# Autodesk Inventor part: ANSI L 3 x 2 x 3_16 00000012
Saved by Autodesk Inventor 2021 (Build 250183000, 183)
## iProperties
Created: 2008-01-07
Part Number: ANSI L 3 x 2 x 3_16 00000012
Material: Generic
Document SubType Name: Modeling
Standard: ANSI
Designer: nino.caldarola
Size Designation: L 3 x 2 x 3/16
Stock Number: L 3 x 2 x 3/16
Density: 1 g/cm^3
Appearance: Default
_FrameMemberDoc: Frame Member File
_Version: 12.0.0
_CCFamilyMember: 5
_CCFamilyDisplayName: ANSI L (Unequal angles) - Angle Steel
G_L: 14.738 in
G_W: 2.000 in
G_H: 3.000 in
+E866665F-DFCD-4B43-A752-D40B89ECAD35+CUTDETAIL1: Miter 67.50 deg
+05D53CF9-7399-4BD2-B0F9-E004F241F57C+CUTDETAIL2: Miter 67.50 deg
Author: nino.caldarola
Autodesk Inventor part; units mm, degrees
ref_plane "Start plane" through (0, 0, -21.042) normal (0, 0, 1) x (1, 0, 0)
ref_plane "End plane" through (0, 0, 353.3115) normal (0, 0, 1) x (1, 0, 0)
sketch "Sketch" plane through (0, 0, 0) normal (0, 0, 1) x (1, 0, 0)
  line L0 (0, 76.2) -> (0, 0)
  line L1 (0, 0) -> (50.8, 0)
  line L2 (50.8, 0) -> (50.8, 2.7625)
  line L3 (48.8, 4.7625) -> (12.6365, 4.7625)
  line L4 (4.7625, 12.6365) -> (4.7625, 74.2)
  line L5 (2.7625, 76.2) -> (0, 76.2)
  line L6 (-7.0414, 0) -> (21.5385, 0) construction
  line L7 (0, -8.0414) -> (0, 34.5385) construction
  arc A0 (4.7625, 12.6365) -> (12.6365, 4.7625) centre (12.6365, 12.6365) ccw
  arc A1 (50.8, 2.7625) -> (48.8, 4.7625) centre (48.8, 2.7625) ccw
  arc A2 (4.7625, 74.2) -> (2.7625, 76.2) centre (2.7625, 74.2) ccw
  line L8 (0, 93.5453) -> (0, -24.9725) construction
  line L9 (-18.6925, 0) -> (62.8653, 0) construction
  point P0 (50.8, 4.7625)
  point P1 (4.7625, 4.7625)
  point P2 (4.7625, 76.2)
  dimension "d12" = 4.7625
  dimension "d13" = 76.2
  dimension "d14" = 50.8
  dimension "d15" = 0
  dimension "d16" = 4.7625
  dimension "d17" = 0
  dimension "d18" = 7.874
  dimension "d19" = 2
  constraints: 16 end point, 6 point on circle, 6 point on line, 6 tangent, 3 centre point, 2 collinear, 2 parallel, 1 equal radius
  measures "d12" distance between parallel lines of L4 L0
  measures "d13" distance of L0.start L1.start
  measures "d14" distance of L1.start L1.end
  measures "d15" distance between parallel lines of L6 L1
  measures "d16" distance between parallel lines of L1 L3
  measures "d17" distance between parallel lines of L7 L0
  measures "d18" radius of A0
  measures "d19" radius of A1
extrude "Body" add sketch "Sketch" along normal up to surface (374.3536 mm away) from surface at -21.042
ref_plane "Work Plane3" through (50.8, 38.1, -21.042) normal (-0.3827, 0, -0.9239) x (-0.9239, 0, 0.3827)
split "Split1" plane through (50.8, 38.1, -21.042) removes the side toward (-0.3827, 0, -0.9239)
ref_plane "Work Plane4" through (50.8, 38.1, 353.3115) normal (-0.3827, 0, 0.9239) x (0.9239, 0, 0.3827)
split "Split2" plane through (50.8, 38.1, 353.3115) removes the side toward (-0.3827, 0, 0.9239)
equation "\"d12\" = G_T"
equation "\"d13\" = G_H"
equation "\"d14\" = G_W"
equation "\"d16\" = G_T"
equation "\"d18\" = G_IR"
equation "\"d4\" = G_L"
equation "\"G_W\" = 50.8"
equation "\"G_H\" = 76.2"
equation "\"G_T\" = 4.7625"
equation "\"G_ER\" = 4.064"
equation "\"G_IR\" = 7.874"
equation "\"G_L\" = B_L + G_OFFSET_START + G_OFFSET_END"
equation "\"ex\" = 0"
equation "\"ey\" = 0"
equation "\"G_OFFSET_START\" = 21.04205"
equation "\"G_OFFSET_END\" = 21.04205"
equation "\"d20\" = -G_OFFSET_START"
equation "\"d21\" = G_OFFSET_END + B_L"
equation "\"B_L\" = 332.26948"
body "Solid1"
